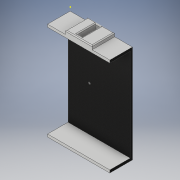
# Autodesk Inventor part: back plate
Saved by Autodesk Inventor 2019 (Build 230136000, 136)
## iProperties
Created: 2020-02-19
Part Number: back plate
Material: Generic
Document SubType Name: Modeling
Designer: LENOVO
Density: 1 g/cm^3
Appearance: Default
Author: LENOVO
Autodesk Inventor part; units mm, degrees
ref_plane "YZ Plane" through (0, 0, 0) normal (1, 0, 0) x (0, 1, 0)
ref_plane "XZ Plane" through (0, 0, 0) normal (0, 1, 0) x (-1, 0, 0)
ref_plane "XY Plane" through (0, 0, 0) normal (0, 0, 1) x (1, 0, 0)
sketch "Sketch1" plane through (0, 0, 0) normal (0, 0, 1) x (1, 0, 0)
  line L0 (0, 0) -> (350, 0)
  line L1 (350, 0) -> (350, 520)
  line L2 (350, 520) -> (0, 520)
  line L3 (0, 520) -> (0, 0)
  dimension "d0" = 350
  dimension "d1" = 520
  constraints: 8 end point, 2 parallel, 1 horizontal, 1 perpendicular
  measures "d0" distance of L2.end L1.end
  measures "d1" distance of L1.end L0.end
extrude "Extrusion1" add sketch "Sketch1" along normal blind 12
sketch "Sketch2" plane through (0, 0, 12) normal (0, 0, 1) x (1, 0, 0)
  line L0 (0, 120) -> (350, 120)
  line L1 (350, 120) -> (350, 370)
  line L2 (350, 0) -> (350, 520) projected
  line L3 (350, 370) -> (0, 370)
  line L4 (0, 520) -> (0, 0) projected
  line L5 (0, 370) -> (0, 520)
  line L6 (350, 520) -> (0, 520) projected
  line L7 (0, 520) -> (350, 520)
  line L8 (350, 520) -> (350, 370)
  circle A0 centre (120, 460) radius 6.5
  circle A1 centre (120, 250) radius 6.5
  dimension "d6" = 13
  dimension "d7" = 13
  constraints: 12 end point, 2 centre point, 2 collinear, 2 perpendicular, 2 point on line, 1 horizontal
  measures "d6" diameter of A0
  measures "d7" diameter of A1
extrude "Extrusion2" cut sketch "Sketch2" against normal blind 12 contours A0 | A1
thread "Thread1" size "M14x2" class "6H" standard "ANSI Metric M Profile" full length
thread "Thread2" size "M14x2" class "6H" standard "ANSI Metric M Profile" full length
sketch "Sketch3" plane through (0, 0, 0) normal (0, 0, -1) x (-1, 0, 0)
  circle A0 centre (-200, 460) radius 6.5
  point P0 (0, 0)
  dimension "d14" = 13
  constraints: 1 centre point
  measures "d14" diameter of A0
extrude "Extrusion3" cut sketch "Sketch3" against normal blind 120
sketch "Sketch4" plane through (0, 520, 0) normal (0, 1, 0) x (1, 0, 0)
  line L0 (0, 0) -> (350, 0) projected
  line L1 (350, 0) -> (350, -12) projected
  line L2 (0, 0) -> (350, 0)
  line L3 (350, 0) -> (350, -12)
  line L4 (350, -12) -> (0, -12)
  line L5 (0, -12) -> (0, 0)
  constraints: 8 end point, 2 parallel, 1 horizontal, 1 perpendicular
extrude "Extrusion4" add sketch "Sketch4" along normal blind 15
sketch "Sketch5" plane through (0, 0, 12) normal (0, 0, 1) x (1, 0, 0)
  line L0 (0, 0) -> (0, 535) projected
  line L1 (0, 535) -> (350, 535)
  line L2 (350, 535) -> (350, 520)
  line L3 (350, 520) -> (0, 520)
  line L4 (0, 520) -> (0, 535)
  dimension "d19" = 350
  dimension "d20" = 15
  constraints: 8 end point, 2 parallel, 1 horizontal, 1 perpendicular
  measures "d19" distance of L2.end L3.end
  measures "d20" distance of L1.end L2.end
extrude "Extrusion5" add sketch "Sketch5" along normal blind 80
sketch "Sketch6" plane through (0, 0, 0) normal (0, -1, 0) x (1, 0, 0)
  line L0 (350, 0) -> (0, 0) projected
  line L1 (350, 12) -> (0, 12) projected
  line L2 (0, 0) -> (350, 0)
  line L3 (350, 0) -> (350, 12)
  line L4 (350, 12) -> (0, 12)
  line L5 (0, 12) -> (0, 0)
  dimension "d23" = 350
  constraints: 8 end point, 2 parallel, 1 horizontal, 1 perpendicular
  measures "d23" distance of L4.end L1.start
extrude "Extrusion6" add sketch "Sketch6" along normal blind 15
sketch "Sketch7" plane through (0, 0, 12) normal (0, 0, 1) x (1, 0, 0)
  line L0 (0, 0) -> (350, 0)
  line L1 (350, 0) -> (350, -15)
  line L2 (350, -15) -> (0, -15)
  line L3 (0, -15) -> (0, 0)
  constraints: 8 end point, 2 parallel, 1 horizontal, 1 perpendicular
extrude "Extrusion7" add sketch "Sketch7" along normal blind 80
sketch "Sketch8" plane through (0, 0, 92) normal (0, 0, 1) x (1, 0, 0)
  line L0 (0, -15) -> (350, -15) projected
  line L1 (0, 0) -> (350, 0)
  line L2 (350, 0) -> (350, -15)
  line L3 (350, -15) -> (0, -15)
  line L4 (0, -15) -> (0, 0)
  line L5 (0, 535) -> (0, 520) projected
  line L6 (0, 520) -> (350, 520) projected
  line L7 (0, 535) -> (350, 535)
  line L8 (350, 535) -> (350, 520)
  line L9 (350, 520) -> (0, 520)
  line L10 (0, 520) -> (0, 535)
  constraints: 16 end point, 4 parallel, 2 horizontal, 2 perpendicular
extrude "Extrusion8" add sketch "Sketch8" along normal blind 35
sketch "Sketch9" plane through (0, -15, 0) normal (0, -1, 0) x (1, 0, 0)
  point P0 (0, 0)
sketch "Sketch10" plane through (0, 535, 0) normal (0, 1, 0) x (1, 0, 0)
  line L0 (0, 0) -> (350, 0) projected
  line L1 (100, 0) -> (250, 0)
  line L2 (250, 0) -> (250, -127)
  line L3 (250, -127) -> (100, -127)
  line L4 (100, -127) -> (100, 0)
  dimension "d30" = 150
  dimension "d31" = 127
  constraints: 8 end point, 2 parallel, 1 horizontal, 1 perpendicular, 1 point on line
  measures "d30" distance of L2.end L3.end
  measures "d31" distance of L1.end L2.end
extrude "Extrusion9" add sketch "Sketch10" along normal blind 20
sketch "Sketch11" plane through (0, 555, 0) normal (0, 1, 0) x (1, 0, 0)
  point P0 (0, 0)
sketch "Sketch12" plane through (0, 555, 0) normal (0, 1, 0) x (1, 0, 0)
  point P0 (0, 0)
sketch "Sketch13" plane through (0, 555, 0) normal (0, 1, 0) x (1, 0, 0)
  line L0 (150, -110) -> (180, -110)
  line L1 (180, -110) -> (180, -10)
  line L2 (180, -10) -> (150, -10)
  line L3 (150, -10) -> (150, -110)
  point P0 (0, 0)
  dimension "d34" = 30
  dimension "d35" = 100
  constraints: 8 end point, 2 parallel, 1 horizontal, 1 perpendicular
  measures "d34" distance of L2.end L1.end
  measures "d35" distance of L1.end L0.end
extrude "Extrusion10" cut sketch "Sketch13" against normal blind 50
fillet "Fillet1" radius 5 8 edges at (180, 555, 60) (150, 555, 60) (165, 555, 110) (165, 555, 10) (175, 555, 127) (250, 555, 63.5) (175, 555, 0) (100, 555, 63.5)
body "Solid1"
